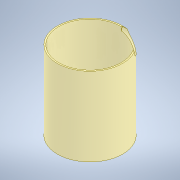
# Autodesk Inventor part: Outside holder
Saved by Autodesk Inventor 2022 (Build 260153000, 153)
## iProperties
Created: 2023-01-18
Part Number: Outside holder
Material: Generic
Document SubType Name: Modeling
Designer: ASUS
Density: 1 g/cm^3
Appearance: Nylon 6
Author: ASUS
Autodesk Inventor part; units mm, degrees
sketch "Sketch1" plane through (0, 0, 0) normal (0, 1, 0) x (-1, 0, 0)
  circle A0 centre (0, 0) radius 36.5
  circle A1 centre (0, 0) radius 35
  dimension "d0" = 73
  dimension "d1" = 70
  constraints: 2 centre point, 2 coincident
  measures "d0" diameter of A0
  measures "d1" diameter of A1
extrude "Extrusion1" add sketch "Sketch1" along normal blind 3 contours A0 | A1
extrude "Extrusion2" add sketch "Sketch1" along normal blind 120
sketch "Sketch2" plane through (0, 3, 0) normal (0, 1, 0) x (1, 0, 0)
  circle A0 centre (0, 0) radius 35 projected
  line L0 (-24.7487, -24.7487) -> (24.7487, -24.7487)
  line L1 (24.7487, -24.7487) -> (24.7487, 24.7487)
  line L2 (24.7487, 24.7487) -> (-24.7487, 24.7487)
  line L3 (-24.7487, 24.7487) -> (-24.7487, -24.7487)
  line L4 (-24.7487, -24.7487) -> (24.7487, 24.7487) construction
  line L5 (24.7487, -24.7487) -> (-24.7487, 24.7487) construction
  constraints: 12 end point, 2 parallel, 1 horizontal, 1 perpendicular, 1 point on circle
extrude "Extrusion3" add sketch "Sketch2" along normal blind 2 contours L1 L0 L3 L2
sketch "Sketch3" plane through (0, 5, 0) normal (0, 1, 0) x (1, 0, 0)
  line L0 (21.1, -23.1) -> (-21.1, -23.1)
  line L1 (-23.1, -21.1) -> (-23.1, 21.1)
  line L2 (-21.1, 23.1) -> (21.1, 23.1)
  line L3 (23.1, 21.1) -> (23.1, -21.1)
  line L4 (23.1, -23.1) -> (-23.1, 23.1) construction
  line L5 (-23.1, -23.1) -> (23.1, 23.1) construction
  arc A0 (-23.1, -21.1) -> (-21.1, -23.1) centre (-21.1, -21.1) ccw
  arc A1 (21.1, -23.1) -> (23.1, -21.1) centre (21.1, -21.1) ccw
  arc A2 (23.1, 21.1) -> (21.1, 23.1) centre (21.1, 21.1) ccw
  arc A3 (-21.1, 23.1) -> (-23.1, 21.1) centre (-21.1, 21.1) ccw
  point P0 (0, 0)
  dimension "d11" = 46.2
  dimension "d12" = 46.2
  dimension "d13" = 2
  constraints: 12 end point, 8 point on circle, 8 point on line, 8 tangent, 4 centre point, 3 equal radius, 2 midpoint, 2 parallel, 1 horizontal, 1 perpendicular
  measures "d11" distance of L4.end L5.end
  measures "d12" distance of L5.start L4.end
  measures "d13" radius of A0
extrude "Extrusion4" cut sketch "Sketch3" against normal blind 2
sketch "Sketch4" plane through (0, 0, 0) normal (1, 0, 0) x (0, 1, 0)
  line L0 (120, 35) -> (120, -35) projected
  line L1 (120, 0) -> (120, -19.5)
  line L2 (120, -19.5) -> (120, -27)
  circle A0 centre (120, -27) radius 9
  point P0 (0, 0)
  dimension "d16" = 19.5
  dimension "d17" = 7.5
  dimension "d18" = 18
  constraints: 4 end point, 2 point on line, 1 centre point, 1 coincident, 1 midpoint
  measures "d16" distance of L1.start L1.end
  measures "d17" distance of L1.end L2.end
  measures "d18" diameter of A0
extrude "Extrusion5" cut sketch "Sketch4" along normal through all
sketch "Sketch5" plane through (0, 0, 0) normal (0, -1, 0) x (1, 0, 0)
  line L0 (5, -36.1559) -> (5, -42.4125)
  line L1 (5, -42.4125) -> (-5, -42.4125)
  line L2 (-5, -42.4125) -> (-5, -36.1559)
  line L3 (-5, -30.5875) -> (5, -42.4125) construction
  line L4 (5, -30.5875) -> (-5, -42.4125) construction
  circle A0 centre (0, 0) radius 36.5 projected
  line L5 (8, -35.6125) -> (8, -42.4125)
  line L6 (8, -42.4125) -> (-8, -42.4125)
  line L7 (-8, -42.4125) -> (-8, -35.6125)
  line L8 (-8, -30.5875) -> (8, -42.4125) construction
  line L9 (8, -30.5875) -> (-8, -42.4125) construction
  circle A1 centre (0, 0) radius 36.5
  arc A2 (5, -36.1675) -> (4.9876, -36.1576) centre (0, -42.4125) ccw
  arc A3 (-4.9876, -36.1576) -> (-5, -36.1675) centre (0, -42.4125) ccw
  arc A4 (-8, -42.4125) -> (8, -42.4125) centre (0, -42.4125) ccw
  arc A5 (-5, -42.4125) -> (5, -42.4125) centre (0, -42.4125) ccw
  point P0 (0, -36.5)
  dimension "d21" = 10
  dimension "d22" = 36.5
  dimension "d23" = 16
  constraints: 20 end point, 14 point on circle, 5 centre point, 5 midpoint, 4 point on line, 2 coincident, 2 parallel
  measures "d21" distance of L1.end L0.end
  measures "d22" distance of A0.centre point (0, -36.5)
  measures "d23" distance of L5.end L6.end
extrude "Extrusion6" add sketch "Sketch5" against normal blind 6 contours A0 L5 L6 L0 | L6 A4 A5 | L6 L7 A0 L2
ref_plane "Work Plane2" through (36.5, 0, 0) normal (1, 0, 0) x (0, 1, 0)
sketch "Sketch8" plane through (36.5, 0, 0) normal (1, 0, 0) x (0, 1, 0)
  line L0 (8.45, 4.25) -> (21.55, 4.25)
  line L1 (21.55, 4.25) -> (21.55, -4.25)
  line L2 (21.55, -4.25) -> (8.45, -4.25)
  line L3 (8.45, -4.25) -> (8.45, 4.25)
  line L4 (8.45, 4.25) -> (21.55, -4.25) construction
  line L5 (21.55, 4.25) -> (8.45, -4.25) construction
  line L6 (7.5, 5.25) -> (22.5, 5.25)
  line L7 (22.5, 5.25) -> (22.5, -5.25)
  line L8 (22.5, -5.25) -> (7.5, -5.25)
  line L9 (7.5, -5.25) -> (7.5, 5.25)
  line L10 (7.5, 5.25) -> (22.5, -5.25) construction
  line L11 (22.5, 5.25) -> (7.5, -5.25) construction
  point P0 (0, 0)
  point P1 (15, 0)
  dimension "d38" = 13.1
  dimension "d39" = 8.5
  dimension "d40" = 0
  dimension "d41" = 15
  dimension "d42" = 10.5
  dimension "d43" = 15
  constraints: 24 end point, 4 midpoint, 4 parallel, 2 horizontal, 2 perpendicular
  measures "d38" distance of L1.end L2.end
  measures "d39" distance of L0.end L1.end
  measures "d40" vertical distance of point (0, 0) point (15, 0)
  measures "d41" distance of point (0, 0) point (15, 0)
  measures "d42" distance of L6.end L7.end
  measures "d43" distance of L7.end L8.end
extrude "Extrusion9" cut sketch "Sketch8" against normal blind 3 contours L0 L1 L2 L3
extrude "Extrusion10" cut sketch "Sketch8" against normal blind 1
ref_plane "Work Plane3" through (0, 93, 0) normal (0, 1, 0) x (1, 0, 0)
ref_plane "Work Plane5" through (0, 32, 0) normal (0, 1, 0) x (1, 0, 0)
sketch "Sketch13" plane through (0, 32, 0) normal (0, 1, 0) x (1, 0, 0)
  circle A0 centre (0, 0) radius 20
  line L0 (24.7487, 24.7487) -> (-24.7487, 24.7487) projected
  circle A1 centre (0, 0) radius 35
  dimension "d61" = 40
  constraints: 2 coincident, 1 centre point, 3 other
  measures "d61" diameter of A0
extrude "Extrusion14" add sketch "Sketch13" along normal blind 3
sketch "Sketch14" plane through (0, 32, 0) normal (0, 1, 0) x (1, 0, 0)
  circle A0 centre (0, 0) radius 50.5551
  constraints: 1 centre point, 1 coincident
extrude "Extrusion15" cut sketch "Sketch14" against normal through all
body "Solid1"
